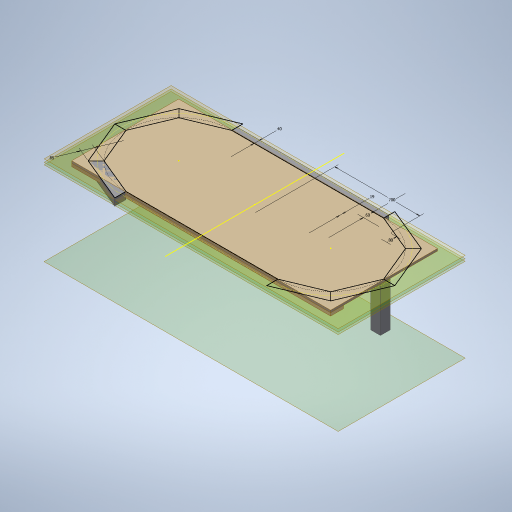
# Autodesk Inventor part: Coposite Top Table Skeleton
Saved by Autodesk Inventor 2024 (Build 280153000, 153)
## iProperties
Category: ESK
Company: UAB Čeli APS
Created: 2008-10-30
Part Number: Coposite Top Table Skeleton
Material: Generic
Description: Stalo eskizas
Document SubType Name: Modeling
Designer: Saulius Dereskeviciu
Mass: 113780 g
Surface Area: 41217.1 cm^2
Volume: 113780 cm^3
Density: 1 g/cm^3
Appearance: Default
Mase: 78.50813211
BetweenInserts: 332,500 mm
InsertN: 3,000 ul
Author: Saulius Dereskeviciu
Autodesk Inventor part; units mm, degrees
ref_plane "YZ Plane" through (0, 0, 0) normal (1, 0, 0) x (0, 1, 0)
ref_plane "XZ Plane" through (0, 0, 0) normal (0, 1, 0) x (-1, 0, 0)
ref_plane "XY Plane" through (0, 0, 0) normal (0, 0, 1) x (1, 0, 0)
sketch "Sketch33" plane through (0, 0, 0) normal (0, 0, 1) x (1, 0, 0)
  line L0 (625, 475) -> (-625, 475)
  line L1 (-625, 475) -> (-625, -475)
  line L2 (-625, -475) -> (625, -475)
  line L3 (625, -475) -> (625, 475)
  circle A0 centre (-625, 0) radius 475
  circle A1 centre (625, 0) radius 475
  line L4 (-1100, 475) -> (1100, 475) construction
  line L5 (1100, 475) -> (1100, -475) construction
  line L6 (1100, -475) -> (-1100, -475) construction
  line L7 (-1100, -475) -> (-1100, 475) construction
  point P0 (0, 0)
  point P1 (0, 475)
  dimension "d88" = 2200
  dimension "d89" = 950
  constraints: 16 end point, 4 horizontal, 4 parallel, 3 midpoint, 3 vertical alignment, 2 perpendicular, 2 vertical, 1 coincident, 1 horizontal alignment, 4 other
  measures "d88" distance of L4.start L4.end
  measures "d89" distance of L6.end L4.start
extrude "Extrusion8" add sketch "Sketch33" along normal blind 60
ref_plane "Inner Layer Top" through (0, 0, 42) normal (0, 0, 1) x (1, 0, 0)
ref_plane "Inner Layer Bottom" through (0, 0, 18) normal (0, 0, -1) x (-1, 0, 0)
sketch "Side Inserts" plane through (0, 0, 60) normal (0, 0, 1) x (1, 0, 0)
  arc A0 (625, -475) -> (625, 475) centre (625, 0) ccw projected
  line L0 (-625, 475) -> (625, 475) projected
  arc A1 (-625, 475) -> (-625, -475) centre (-625, 0) ccw projected
  line L1 (625, -475) -> (-625, -475) projected
  arc A2 (-625, 435) -> (-625, -435) centre (-625, 0) ccw
  line L2 (-625, 435) -> (625, 435)
  arc A3 (625, -435) -> (625, 435) centre (625, 0) ccw
  line L3 (625, -435) -> (-625, -435)
  line L4 (-1065, 440) -> (1065, 440)
  line L5 (1065, 440) -> (1065, 335)
  line L6 (1065, 335) -> (-1065, 335)
  line L7 (-1065, 335) -> (-1065, 440)
  line L8 (-1060, 503.9834) -> (-1060, -438.8522) construction
  line L9 (-1612.8047, 0) -> (1612.8047, 0) projected
  line L10 (-625, -435) -> (625, -435)
  line L11 (-1065, -440) -> (1065, -440)
  line L12 (1065, -440) -> (1065, -335)
  line L13 (1065, -335) -> (-1065, -335)
  line L14 (-1065, -335) -> (-1065, -440)
  point P0 (0, 0)
  point P1 (0, 335)
  point P2 (0, -335)
  dimension "d94" = 40
  dimension "d95" = 5
  dimension "d96" = 100
  dimension "d97" = 5
  constraints: 24 end point, 5 symmetric about line, 4 point on circle, 3 parallel, 2 centre point, 1 horizontal, 1 midpoint, 1 perpendicular, 1 tangent, 1 vertical alignment, 3 other
  measures "d94" distance between parallel lines of L0 L2
  measures "d95" distance between parallel lines of L2 L4
  measures "d96" distance between parallel lines of L6 L2
  measures "d97" distance between parallel lines of L8 L7
extrude "Extrusion9" add sketch "Side Inserts" against normal up to surface (24 mm away) from surface at -18 separate body contours L11 A1 L13 A2 L3 A3 A0 | A0 L13 L12 L11 | L11 L14 L13 A1 | A3 L3 A2 L13
sketch "Top&Bottom Plate" plane through (0, 0, 60) normal (0, 0, 1) x (1, 0, 0)
  arc A0 (-625, 475) -> (-625, -475) centre (-625, 0) ccw projected
  line L0 (-1065, 440) -> (1065, 440)
  line L1 (1065, 440) -> (1065, -440)
  line L2 (1065, -440) -> (-1065, -440)
  line L3 (-1065, -440) -> (-1065, 440)
  point P0 (0, 0)
  point P1 (0, -440)
  point P2 (-1100, 0)
  point P3 (-1065, 0)
  constraints: 8 end point, 2 horizontal alignment, 2 midpoint, 2 parallel, 1 coincident, 1 horizontal, 1 perpendicular, 1 point on circle, 1 vertical alignment
extrude "Extrusion10" add sketch "Top&Bottom Plate" against normal up to surface (18 mm away) separate body contours L0 L1 L2 A0 L3 | A0 L3 L0 | A0 L2 L3
sketch "Timber Frame" plane through (0, 0, 60) normal (0, 0, 1) x (1, 0, 0)
  arc A0 (625, -475) -> (625, 475) centre (625, 0) ccw construction
  line L0 (-625, 475) -> (625, 475) construction
  arc A1 (-625, 475) -> (-625, -475) centre (-625, 0) ccw construction
  line L1 (625, -475) -> (-625, -475) construction
  arc A2 (-625, 435) -> (-625, -435) centre (-625, 0) ccw construction
  line L2 (-625, 435) -> (625, 435)
  arc A3 (625, -435) -> (625, 435) centre (625, 0) ccw construction
  line L3 (625, -435) -> (-625, -435)
  line L4 (-625, -435) -> (-932.5914, -307.5914)
  line L5 (-932.5914, -307.5914) -> (-1060, 0)
  line L6 (-1060, 0) -> (-932.5914, 307.5914)
  line L7 (-932.5914, 307.5914) -> (-625, 435)
  line L8 (-625, -527.0033) -> (-997.6476, -372.6476)
  line L9 (-997.6476, -372.6476) -> (-1152.0033, 0)
  line L10 (-1152.0033, 0) -> (-997.6476, 372.6476)
  line L11 (-997.6476, 372.6476) -> (-625, 527.0033)
  line L12 (-625, 435) -> (-625, 527.0033)
  line L13 (-625, -435) -> (-625, -527.0033)
  line L14 (-932.5914, 307.5914) -> (-997.6476, 372.6476)
  line L15 (-1060, 0) -> (-1152.0033, 0)
  line L16 (-932.5914, -307.5914) -> (-997.6476, -372.6476)
  line L17 (0, -737.8047) -> (0, 737.8047) projected
  line L18 (625, -435) -> (932.5914, -307.5914)
  line L19 (932.5914, -307.5914) -> (1060, 0)
  line L20 (1060, 0) -> (932.5914, 307.5914)
  line L21 (932.5914, 307.5914) -> (625, 435)
  line L22 (625, -527.0033) -> (997.6476, -372.6476)
  line L23 (997.6476, -372.6476) -> (1152.0033, 0)
  line L24 (1152.0033, 0) -> (997.6476, 372.6476)
  line L25 (997.6476, 372.6476) -> (625, 527.0033)
  line L26 (625, 435) -> (625, 527.0033)
  line L27 (625, -435) -> (625, -527.0033)
  line L28 (932.5914, 307.5914) -> (997.6476, 372.6476)
  line L29 (1060, 0) -> (1152.0033, 0)
  line L30 (932.5914, -307.5914) -> (997.6476, -372.6476)
  line L31 (-625, 435) -> (625, 435) construction
  line L32 (-625, -435) -> (625, -435) construction
  point P0 (0, 0)
  dimension "d98" = 40
  dimension "d99" = 85
  constraints: 60 end point, 11 symmetric about line, 8 point on circle, 5 parallel, 4 equal length, 4 tangent, 2 centre point, 2 collinear, 2 horizontal alignment, 1 perpendicular, 1 vertical alignment, 3 other
  measures "d98" distance between parallel lines of L0 L2
  measures "d99" distance between parallel lines of L8 L4
extrude "Extrusion11" add sketch "Timber Frame" against normal up to surface (60 mm away) separate body contours L13 L8 L16 L4
sketch "Inner Inserts" plane through (0, 0, 60) normal (0, 0, 1) x (1, 0, 0)
  line L0 (-1065, -440) -> (-1065, 440) projected
  line L1 (1065, 335) -> (-1065, 335) construction
  line L2 (1065, 440) -> (1065, -440) projected
  line L3 (1065, -335) -> (-1065, -335) construction
  line L4 (-1065, 335) -> (-665, 335)
  line L5 (-665, 335) -> (-665, -335)
  line L6 (-665, -335) -> (-1065, -335)
  line L7 (-1065, -335) -> (-1065, 335)
  line L8 (-302.5, 335) -> (-362.5, 335)
  line L9 (-362.5, 335) -> (-362.5, -335)
  line L10 (-362.5, -335) -> (-302.5, -335)
  line L11 (-302.5, -335) -> (-302.5, 335)
  line L12 (1065, 335) -> (665, 335) construction
  line L13 (665, 335) -> (665, -335) construction
  line L14 (665, -335) -> (1065, -335) construction
  line L15 (1065, -335) -> (1065, 335) construction
  line L16 (-332.5, 335) -> (-332.5, -335) construction
  line L17 (30, -335) -> (30, 335)
  line L18 (0, 335) -> (0, -335) construction
  line L19 (-30, -335) -> (30, -335)
  line L20 (30, 335) -> (-30, 335)
  line L21 (-30, 335) -> (-30, -335)
  line L22 (362.5, -335) -> (362.5, 335)
  line L23 (332.5, 335) -> (332.5, -335) construction
  line L24 (302.5, -335) -> (362.5, -335)
  line L25 (362.5, 335) -> (302.5, 335)
  line L26 (302.5, 335) -> (302.5, -335)
  point P0 (0, 0)
  dimension "InsertN" = 3
  dimension "d100" = 400
  dimension "d101" = 60
  dimension "IsertsSpace" = 1330
  dimension "BetweenInserts" = 332.5
  dimension "d124" = 332.5
  constraints: 46 end point, 6 parallel, 4 collinear, 4 horizontal, 3 perpendicular, 3 point on line, 2 midpoint, 22 other
  measures "d100" distance of L1.end L4.end
  measures "d101" distance of L8.start L8.end
  measures "IsertsSpace" distance between parallel lines of L13 L5
  measures "BetweenInserts" distance between parallel lines of L16 L5
  measures "d124" distance of L10.end L17.start
extrude "Extrusion12" add sketch "Inner Inserts" along normal up to surface (24 mm away) from surface at -42 separate body contours L0 L4 L5 L6
extrude "Extrusion13" add sketch "Inner Inserts" against normal up to surface (24 mm away) from surface at -18 separate body contours L11 L10 L9 L8
ref_plane "Bottom Plane" through (0, 0, 0) normal (0, 0, -1) x (-1, 0, 0)
sketch "Insert Along Edge" plane through (0, 0, 60) normal (0, 0, 1) x (1, 0, 0)
  line L0 (-625, 475) -> (625, 475) projected
  line L1 (-625, 435) -> (-625, 527.0033) construction
  line L2 (625, 435) -> (625, 527.0033) construction
  line L3 (-625, 435) -> (625, 435)
  line L4 (625, 435) -> (625, 480)
  line L5 (625, 480) -> (-625, 480)
  line L6 (-625, 480) -> (-625, 435)
  point P0 (0, 0)
  dimension "d104" = 5
  constraints: 8 end point, 2 parallel, 1 horizontal, 1 perpendicular, 1 point on line
  measures "d104" distance between parallel lines of L0 L5
extrude "Extrusion14" add sketch "Insert Along Edge" against normal up to surface (60 mm away) separate body
sketch "Outside Contour of table" plane through (0, 0, 60) normal (0, 0, 1) x (1, 0, 0)
  arc A0 (625, -475) -> (625, 475) centre (625, 0) ccw projected
  line L0 (-625, 475) -> (625, 475) projected
  arc A1 (-625, 475) -> (-625, -475) centre (-625, 0) ccw projected
  line L1 (625, -475) -> (-625, -475) projected
  point P0 (0, 0)
sketch "Legs position" plane through (0, 0, 0) normal (0, 0, -1) x (-1, 0, 0)
  line L0 (-625, 475) -> (625, 475) projected
  line L1 (-620, 335) -> (620, 335)
  line L2 (620, 335) -> (620, -335)
  line L3 (620, -335) -> (-620, -335)
  line L4 (-620, -335) -> (-620, 335)
  line L5 (639, 354) -> (-639, 354)
  line L6 (-639, 354) -> (-639, -354)
  line L7 (-639, -354) -> (639, -354)
  line L8 (639, -354) -> (639, 354)
  line L9 (-620, 335) -> (-700, 335)
  line L10 (-700, 335) -> (-700, 415)
  line L11 (-700, 415) -> (-620, 415)
  line L12 (-620, 415) -> (-620, 335)
  line L13 (-620, -335) -> (-639, -335)
  line L14 (620, 335) -> (620, 354)
  line L15 (-620, 335) -> (-639, 335)
  line L16 (-620, 335) -> (-620, 354)
  point P0 (0, 0)
  point P1 (-620, 0)
  point P2 (0, 335)
  dimension "d105" = 19
  dimension "d106" = 80
  dimension "d107" = 60
  dimension "d108" = 700
  constraints: 32 end point, 6 parallel, 6 perpendicular, 6 point on line, 2 horizontal, 2 midpoint, 1 horizontal alignment, 1 vertical alignment, 3 other
  measures "d105" distance between parallel lines of L1 L5
  measures "d106" distance of L9.end L10.end
  measures "d107" distance between parallel lines of L0 L11
  measures "d108" distance from line of L10 point (0, 0)
ref_plane "Bottom of leg" through (0, 0, -690) normal (0, 0, -1) x (-1, 0, 0)
extrude "Extrusion15" add sketch "Legs position" along normal up to surface (690 mm away) separate body contours L9 L6 L5 L12 | L9 L10 L11 L12 L5 L6
sketch "Sketch41" plane through (0, 0, 0) normal (0, 0, 1) x (1, 0, 0)
  circle A0 centre (660, 375) radius 25
  line L0 (620, 415) -> (620, 335) projected
  line L1 (700, 415) -> (620, 415) projected
  point P0 (0, 0)
  point P1 (620, 375)
  point P2 (660, 415)
  dimension "d133" = 50
  constraints: 2 midpoint, 1 centre point, 1 horizontal alignment, 1 vertical alignment
  measures "d133" diameter of A0
extrude "Extrusion16" add sketch "Sketch41" along normal blind 40 and the other way blind 100 separate body
extrude "Extrusion17" add sketch "Legs position" along normal blind 80 separate body contours L4 L13 L6 L9
extrude "Extrusion18" add sketch "Legs position" along normal up to surface (80 mm away) separate body contours L12 L5 L14 L1
equation "\"InsertN\" = 3"
equation "\"d124\" = BetweenInserts"
